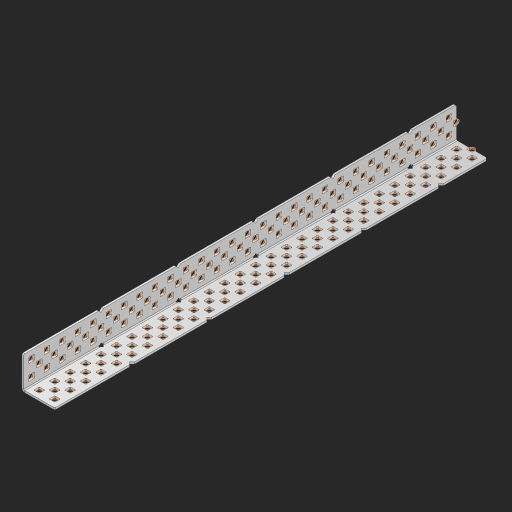
# Autodesk Inventor part: Alu C 1x2x1x35
Saved by Autodesk Inventor 2023 (Build 270158000, 158)
## iProperties
Created: 2022-07-28
Part Number: Alu C 1x2x1x35
Material: Generic
Document SubType Name: Sheet Metal
Designer: ylu12
Density: 1 g/cm^3
Sheet Metal Rule: Default
Appearance: Aluminum
Author: ylu12
Autodesk Inventor part; units mm, degrees
ref_plane "YZ Plane" through (0, 0, 0) normal (1, 0, 0) x (0, 1, 0)
ref_plane "XZ Plane" through (0, 0, 0) normal (0, 1, 0) x (-1, 0, 0)
sketch "Sketch1" plane through (0, 0, 0) normal (0, 1, 0) x (-1, 0, 0)
  line L0 (-12.7, 0) -> (12.7, 0)
  line L1 (12.7, 0) -> (12.7, -355.6)
  line L2 (12.7, -355.6) -> (-12.7, -355.6)
  line L3 (-12.7, -355.6) -> (-12.7, 0)
  line L4 (12.7, 0) -> (-12.7, -355.6) construction
  point P0 (0, 0)
  point P1 (0, 0)
  dimension "d0" = 25.4
  dimension "d1" = 355.6
  measures "d0" distance of L1.end L2.end
  measures "d1" distance of L0.end L1.end
extrude "Plate1" add sketch "Sketch1" along normal blind 1.5875
sketch "Sketch2" plane through (-12.7, 1.5875, 0) normal (-1, 0, 0) x (0, -1, 0)
  line L0 (0, -355.6) -> (0, 0)
  line L1 (0, 0) -> (-25.4, 0)
  line L2 (-25.4, 0) -> (-25.4, -355.6)
  line L3 (-25.4, -355.6) -> (0, -355.6)
  constraints: 6 end point, 1 horizontal, 1 perpendicular, 1 vertical
edge flange "Flanges" height 25.4 angle 90 thickness 1.5875 bend radius 0.7937 thickness toward (-1, 0, 0) relief tear relief width 1.5875 relief depth 0.7937 edges at (-12.7, 1.5875, -177.8) wall of the first edge with corners at (-12.7, 1.5875, -355.6) (-12.7, 1.5875, 0) (-12.7, 26.9875, 0) (-12.7, 26.9875, -355.6)
bend "Bend1"
corner "Corner1"
sketch "Sketch8" plane through (0, 0, 0) normal (0, -1, 0) x (1, 0, 0)
  line L0 (12.7, 0) -> (-11.9062, 0) construction
  line L1 (8.1534, -4.0386) -> (4.5466, -4.0386)
  line L2 (4.0386, -4.5466) -> (4.0386, -8.1534)
  line L3 (4.5466, -8.6614) -> (8.1534, -8.6614)
  line L4 (8.6614, -8.1534) -> (8.6614, -4.5466)
  arc A0 (8.6614, -4.5466) -> (8.1534, -4.0386) centre (8.1534, -4.5466) ccw
  arc A1 (8.1534, -8.6614) -> (8.6614, -8.1534) centre (8.1534, -8.1534) ccw
  arc A2 (4.0386, -8.1534) -> (4.5466, -8.6614) centre (4.5466, -8.1534) ccw
  arc A3 (4.5466, -4.0386) -> (4.0386, -4.5466) centre (4.5466, -4.5466) ccw
  line L5 (8.1534, -4.5466) -> (4.5466, -8.1534) construction
  line L6 (12.7, -355.6) -> (12.7, 0) construction
  point P0 (0, 0)
  point P1 (4.0386, -8.6614)
  point P2 (8.6614, -8.6614)
  point P3 (6.35, -6.35)
  dimension "d49" = 4.6228
  dimension "d50" = 0.508
  dimension "d52" = 6.35
  dimension "d123" = 6.35
  constraints: 10 end point, 8 point on circle, 8 tangent, 4 centre point, 4 point on line, 3 equal radius, 2 parallel, 2 perpendicular, 1 horizontal, 1 midpoint
  measures "d49" distance of point (8.661, -8.661) point (4.039, -8.661)
  measures "d50" radius of A0
  measures "d52" distance from line of L0 point (6.35, -6.35)
  measures "d123" distance from line of L6 point (6.35, -6.35)
extrude "Body Stamp" cut sketch "Sketch8" against normal blind 1.5875
sketch "Sketch9" plane through (0, 0, 0) normal (0, -1, 0) x (1, 0, 0)
  arc A0 (8.6614, -4.5466) -> (8.1534, -4.0386) centre (8.1534, -4.5466) ccw construction
  arc A1 (4.0386, -8.1534) -> (4.5466, -8.6614) centre (4.5466, -8.1534) ccw construction
  line L0 (8.1534, -4.5466) -> (4.5466, -8.1534) construction
  circle A2 centre (6.35, -6.35) radius 2.1844
  point P0 (0, 0)
  dimension "d55" = 4.3688
  constraints: 2 end point, 1 centre point, 1 midpoint
  measures "d55" diameter of A2
surface extrude "Body Circle" sketch "Sketch9" against normal up to surface (1.5875 mm away) shown yes curves A2
pattern_sketch "Body Pattern" of "Body Stamp", "Body Circle" from (6.35, 0, -6.35) copies at (6.35, 0, -19.05) at (6.35, 0, -31.75) at (6.35, 0, -44.45) at (-6.35, 0, -6.35) at (-6.35, 0, -19.05) at (-6.35, 0, -31.75) at (-6.35, 0, -44.45) at (6.35, 0, -57.15) at (-6.35, 0, -57.15) at (6.35, 0, -69.85) at (-6.35, 0, -69.85) at (6.35, 0, -82.55) at (-6.35, 0, -82.55) at (6.35, 0, -95.25) at (-6.35, 0, -95.25) at (6.35, 0, -107.95) at (-6.35, 0, -107.95) at (6.35, 0, -120.65) at (-6.35, 0, -120.65) at (6.35, 0, -133.35) at (-6.35, 0, -133.35) at (6.35, 0, -146.05) at (-6.35, 0, -146.05) at (6.35, 0, -158.75) at (-6.35, 0, -158.75) at (6.35, 0, -171.45) at (-6.35, 0, -171.45) at (6.35, 0, -184.15) at (-6.35, 0, -184.15) at (6.35, 0, -196.85) at (-6.35, 0, -196.85) at (6.35, 0, -209.55) at (-6.35, 0, -209.55) at (6.35, 0, -222.25) at (-6.35, 0, -222.25) at (6.35, 0, -234.95) at (-6.35, 0, -234.95) at (6.35, 0, -247.65) at (-6.35, 0, -247.65) at (6.35, 0, -260.35) at (-6.35, 0, -260.35) at (6.35, 0, -273.05) at (-6.35, 0, -273.05) at (6.35, 0, -285.75) at (-6.35, 0, -285.75) at (6.35, 0, -298.45) at (-6.35, 0, -298.45) at (6.35, 0, -311.15) at (-6.35, 0, -311.15) at (6.35, 0, -323.85) at (-6.35, 0, -323.85) at (6.35, 0, -336.55) at (-6.35, 0, -336.55) at (6.35, 0, -349.25) at (-6.35, 0, -349.25)
sketch "Sketch15" plane through (0, 0, 0) normal (0, -1, 0) x (1, 0, 0)
  line L0 (12.7, 0) -> (-11.9062, 0) construction
  line L1 (1.8034, -10.3886) -> (-1.8034, -10.3886)
  line L2 (-2.3114, -10.8966) -> (-2.3114, -14.5034)
  line L3 (-1.8034, -15.0114) -> (1.8034, -15.0114)
  line L4 (2.3114, -14.5034) -> (2.3114, -10.8966)
  arc A0 (2.3114, -10.8966) -> (1.8034, -10.3886) centre (1.8034, -10.8966) ccw
  arc A1 (1.8034, -15.0114) -> (2.3114, -14.5034) centre (1.8034, -14.5034) ccw
  arc A2 (-1.8034, -10.3886) -> (-2.3114, -10.8966) centre (-1.8034, -10.8966) ccw
  arc A3 (-2.3114, -14.5034) -> (-1.8034, -15.0114) centre (-1.8034, -14.5034) ccw
  line L5 (1.8034, -10.8966) -> (-1.8034, -14.5034) construction
  line L6 (12.7, 0) -> (12.7, -444.5) construction
  line L7 (0, 0) -> (0, -12.7) construction
  point P0 (10.3187, 0)
  point P1 (-2.3114, -15.0114)
  point P2 (2.3114, -15.0114)
  dimension "d106" = 4.6228
  dimension "d107" = 0.508
  dimension "d108" = 12.7
  constraints: 12 end point, 8 point on circle, 8 tangent, 4 centre point, 4 point on line, 3 equal radius, 2 parallel, 2 perpendicular, 1 horizontal, 1 midpoint, 1 vertical
  measures "d106" distance of point (2.311, -15.011) point (-2.311, -15.011)
  measures "d107" radius of A0
  measures "d108" distance from line of L0 L7.end
extrude "Center Stamp" cut sketch "Sketch15" against normal blind 1.5875
sketch "Sketch16" plane through (0, 0, 0) normal (0, -1, 0) x (1, 0, 0)
  circle A0 centre (0, -12.7) radius 2.1844
  line L0 (12.7, 0) -> (12.7, -444.5) construction
  arc A1 (-1.8034, -10.3886) -> (-2.3114, -10.8966) centre (-1.8034, -10.8966) ccw construction
  arc A2 (1.8034, -15.0114) -> (2.3114, -14.5034) centre (1.8034, -14.5034) ccw construction
  line L1 (-1.8034, -10.8966) -> (1.8034, -14.5034) construction
  point P0 (0, 0)
  point P1 (10.3187, 0)
  dimension "d112" = 4.3688
  constraints: 2 end point, 1 centre point, 1 coincident, 1 midpoint
  measures "d112" diameter of A0
surface extrude "Center Circle" sketch "Sketch16" against normal up to surface (1.5875 mm away) shown yes curves A0
pattern_linear "Center Pattern" count 28 spacing 12.7 along (0, 0, -1) of "Center Circle", "Center Stamp"
sketch "Arc Length" plane through (11.1125, 2.3812, 0) normal (0, 0, 1) x (1, 0, 0)
  line L0 (-25.4, 0) -> (-23.8125, 0) projected
  arc A0 (-25.4, 0) -> (-23.0187, -2.3813) centre (-23.0187, 0) ccw projected
  line L1 (-23.0187, -0.7938) -> (-23.0187, -2.3813) projected
  arc A1 (-23.8125, 0) -> (-23.0187, -0.7938) centre (-23.0187, 0) ccw projected
  point P0 (-11.1125, -2.3812)
  dimension "d126" = 1.2468
  dimension "d127" = 3.7405
sketch "Sketch13" plane through (-14.2875, 14.2875, 88.9) normal (1, 0, 0) x (0, 0, -1)
  line L0 (150.368, 12.7) -> (152.4, 10.668)
  line L1 (152.4, 10.668) -> (154.432, 12.7)
  line L2 (150.368, 12.7) -> (154.432, 12.7)
  line L3 (152.4, -10.8903) -> (150.1372, -13.1531)
  line L4 (150.1372, -13.1531) -> (152.4, -15.4159)
  line L5 (152.4, -15.4159) -> (154.6628, -13.1531)
  line L6 (154.6628, -13.1531) -> (152.4, -10.8903)
  line L7 (152.4, -10.8903) -> (152.4, -15.4159) construction
  line L8 (152.4, 10.668) -> (152.4, -10.8903) construction
  line L9 (444.5, 12.7) -> (88.9, 12.7) projected
  line L10 (444.5, -11.9062) -> (88.9, -11.9062) construction
  line L11 (88.9, 12.7) -> (88.9, -11.9062) construction
  point P0 (88.9, -14.2875)
  dimension "d86" = 4.5256
  dimension "d128" = 2.032
  dimension "d129" = 1.016
  dimension "d130" = 63.5
  constraints: 19 end point, 6 perpendicular, 2 vertical, 1 collinear
  measures "d86" distance of L3.start L4.end
  measures "d128" distance from line of L2 L0.end
  measures "d129" distance from line of L3.start L10
  measures "d130" distance between parallel lines of L11 L8
cut across bends "Notch" sketch "Sketch13" k factor 0.44
pattern_linear "Notch Pattern" count 5 spacing 63.5 along (0, 0, -1) of "Notch"
ref_plane "Diagonal Plane" through (-12.7, 1.5875, 0) normal (-0.7071068, 0.7071068, 0) x (0, 0, 1)
mirror "Everything Mirrored" about plane through (-12.7, 1.5875, 0) normal (-0.7071068, 0.7071068, 0) of "Body Stamp", "Body Circle", "Body Pattern", "Center Stamp", "Center Circle", "Center Pattern", "Notch", "Notch Pattern"
chamfer "End Chamfer" distance 1.016 angle 45 4 edges at (-13.4937, 26.9875, -355.6) (-13.4937, 26.9875, 0) (12.7, 0.7937, 0) (12.7, 0.7937, -355.6)
sketch "Body Pattern Sketch" plane through (0, 0, 0) normal (0, -1, 0) x (1, 0, 0)
  line L0 (12.7, 0) -> (-11.9062, 0) construction
  line L1 (12.7, 0) -> (12.7, -444.5) construction
  point P0 (0, 0)
  point P1 (6.35, -6.35)
  point P2 (6.35, -19.05)
  point P3 (6.35, -31.75)
  point P4 (6.35, -44.45)
  point P5 (-6.35, -6.35)
  point P6 (-6.35, -19.05)
  point P7 (-6.35, -31.75)
  point P8 (-6.35, -44.45)
  point P9 (6.35, -57.15)
  point P10 (-6.35, -57.15)
  point P11 (6.35, -69.85)
  point P12 (-6.35, -69.85)
  point P13 (6.35, -82.55)
  point P14 (-6.35, -82.55)
  point P15 (6.35, -95.25)
  point P16 (-6.35, -95.25)
  point P17 (6.35, -107.95)
  point P18 (-6.35, -107.95)
  point P19 (6.35, -120.65)
  point P20 (-6.35, -120.65)
  point P21 (6.35, -133.35)
  point P22 (-6.35, -133.35)
  point P23 (6.35, -146.05)
  point P24 (-6.35, -146.05)
  point P25 (6.35, -158.75)
  point P26 (-6.35, -158.75)
  point P27 (6.35, -171.45)
  point P28 (-6.35, -171.45)
  point P29 (6.35, -184.15)
  point P30 (-6.35, -184.15)
  point P31 (6.35, -196.85)
  point P32 (-6.35, -196.85)
  point P33 (6.35, -209.55)
  point P34 (-6.35, -209.55)
  point P35 (6.35, -222.25)
  point P36 (-6.35, -222.25)
  point P37 (6.35, -234.95)
  point P38 (-6.35, -234.95)
  point P39 (6.35, -247.65)
  point P40 (-6.35, -247.65)
  point P41 (6.35, -260.35)
  point P42 (-6.35, -260.35)
  point P43 (6.35, -273.05)
  point P44 (-6.35, -273.05)
  point P45 (6.35, -285.75)
  point P46 (-6.35, -285.75)
  point P47 (6.35, -298.45)
  point P48 (-6.35, -298.45)
  point P49 (6.35, -311.15)
  point P50 (-6.35, -311.15)
  point P51 (6.35, -323.85)
  point P52 (-6.35, -323.85)
  point P53 (6.35, -336.55)
  point P54 (-6.35, -336.55)
  point P55 (6.35, -349.25)
  point P56 (-6.35, -349.25)
  dimension "d62" = 12.7
  dimension "d65" = 12.7
  dimension "d99" = 6.35
  dimension "d125" = 6.35
  constraints: 1 horizontal, 1 vertical, 55 other
  measures "d99" distance from line of L0 point (6.35, -6.35)
  measures "d125" horizontal distance of point (0, 0) point (6.35, -6.35)
equation "\"d1\" = 12.7 * Length"
equation "\"d53\" = Thickness"
equation "\"d89\" = Thickness"
equation "\"d2\" = Thickness"
equation "\"d3\" = BendReliefWidth"
equation "\"d4\" = BendReliefDepth"
equation "\"d5\" = MinimumRemnant"
equation "\"d6\" = TransitionRadius"
equation "\"d10\" = CornerReliefSize"
equation "\"d11\" = GapSize"
equation "\"d12\" = JacobiRadiusSize"
equation "\"BendRadius\" = Thickness"
equation "\"BendReliefWidth\" = Thickness"
equation "\"BendReliefDepth\" = 0.5 * Thickness"
equation "\"CornerReliefSize\" = 4 * Thickness"
equation "\"MinimumRemnant\" = 2 * Thickness"
equation "\"TransitionRadius\" = BendRadius"
equation "\"JacobiRadiusSize\" = BendRadius"
equation "\"GapSize\" = Thickness"
equation "\"Length\" = 28"
equation "\"Thickness\" = 1.5875"
body "Solid1"
body "Srf91"
body "Srf92"
body "Srf786"
body "Srf856"
body "Srf857"
body "Srf858"
body "Srf859"
body "Srf860"
body "Srf861"
body "Srf889"
body "Srf890"
body "Srf891"
body "Srf1275"
body "Srf1276"
body "Srf1278"
body "Srf1279"
body "Srf1280"
body "Srf1281"
body "Srf1282"
body "Srf1283"
body "Srf1277"
body "Srf1285"
body "Srf1286"
body "Srf1287"
body "Srf1383"
body "Srf1384"
body "Srf1385"
body "Srf1386"
body "Srf1387"
body "Srf1388"
body "Srf1389"
body "Srf1390"
body "Srf1391"
body "Srf1392"
body "Srf1393"
body "Srf1394"
body "Srf1395"
body "Srf1396"
body "Srf1397"
body "Srf1398"
body "Srf1399"
body "Srf1400"
body "Srf1401"
body "Srf1402"
body "Srf1403"
body "Srf1404"
body "Srf1405"
body "Srf1406"
body "Srf1407"
body "Srf1408"
body "Srf1409"
body "Srf1410"
body "Srf1411"
body "Srf1412"
body "Srf1413"
body "Srf1414"
body "Srf1415"
body "Srf1416"
body "Srf1417"
body "Srf1418"
body "Srf1419"
body "Srf1420"
body "Srf1421"
body "Srf1422"
body "Srf1423"
body "Srf1424"
body "Srf1425"
body "Srf1426"
body "Srf1427"
body "Srf1428"
body "Srf1429"
body "Srf1430"
body "Srf1445"
body "Srf1446"
body "Srf1447"
body "Srf1448"
body "Srf1449"
body "Srf1450"
body "Srf1451"
body "Srf1452"
body "Srf1453"
body "Srf1454"
body "Srf1455"
body "Srf1456"
body "Srf1457"
body "Srf1458"
body "Srf1459"
body "Srf1460"
body "Srf1461"
body "Srf1462"
body "Srf1463"
body "Srf1464"
body "Srf1465"
body "Srf1466"
body "Srf1467"
body "Srf1468"
body "Srf1475"
body "Srf1476"
body "Srf1477"
body "Srf1478"
body "Srf1479"
body "Srf1480"
body "Srf1481"
body "Srf1482"
body "Srf1483"
body "Srf1484"
body "Srf1485"
body "Srf1486"
body "Srf1487"
body "Srf1488"
body "Srf1489"
body "Srf1490"
body "Srf1491"
body "Srf1492"
body "Srf1493"
body "Srf1494"
body "Srf1495"
body "Srf1496"
body "Srf1497"
body "Srf1498"
body "Srf1499"
body "Srf1500" dims "d2" = 1.5875 (= Thickness), "d10" = 6.35 (= CornerReliefSize)
body "Srf1501"
body "Srf1502"
body "Srf1503"
body "Srf1504"
body "Srf1505"
body "Srf1506"
body "Srf1507"
body "Srf1508"
body "Srf1509"
body "Srf1510"
body "Srf1511"
body "Srf1512"
body "Srf1513"
body "Srf1514"
body "Srf1515"
body "Srf1516"
body "Srf1517"
body "Srf1518"
body "Srf1519"
body "Srf1520"
body "Srf1521"
body "Srf1522"
body "Srf1537"
body "Srf1538"
body "Srf1539"
body "Srf1540"
body "Srf1541"
body "Srf1542"
body "Srf1543"
body "Srf1544"
body "Srf1545"
body "Srf1546"
body "Srf1547"
body "Srf1548"
body "Srf1549"
body "Srf1550"
body "Srf1551"
body "Srf1552"
body "Srf1553"
body "Srf1554"
body "Srf1555"
body "Srf1556"
body "Srf1557"
body "Srf1558"
body "Srf1559"
body "Srf1560"
